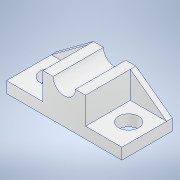
# Autodesk Inventor part: Part1
Saved by Autodesk Inventor 2022 (Build 260153000, 153)
## iProperties
Created: 2021-10-05
Part Number: Part1
Material: Aluminum 6061
Document SubType Name: Modeling
Designer: Lucas
Density: 2.7 g/cm^3
Appearance: Aluminum - Flat
Mass: 213.769 g
Surface Area: 180.738 cm^2
Volume: 79.1737 cm^3
Author: Lucas
Autodesk Inventor part; units mm, degrees
ref_plane "YZ Plane" through (0, 0, 0) normal (1, 0, 0) x (0, 1, 0)
ref_plane "XZ Plane" through (0, 0, 0) normal (0, 1, 0) x (-1, 0, 0)
ref_plane "XY Plane" through (0, 0, 0) normal (0, 0, 1) x (1, 0, 0)
sketch "Sketch1" plane through (0, 0, 0) normal (0, 0, 1) x (1, 0, 0)
  line L0 (-51.5, 0) -> (51.5, 0)
  line L1 (51.5, 0) -> (51.5, 10)
  line L2 (51.5, 10) -> (19, 10)
  line L3 (19, 10) -> (19, 34)
  line L4 (19, 34) -> (10, 34)
  arc A0 (-10, 34) -> (10, 34) centre (0, 34) ccw
  line L5 (-10, 34) -> (-19, 34)
  line L6 (-19, 34) -> (-19, 10)
  line L7 (-19, 10) -> (-51.5, 10)
  line L8 (-51.5, 10) -> (-51.5, 0)
  point P0 (0, 0)
  dimension "d0" = 103
  dimension "d4" = 38
  dimension "d6" = 34
  dimension "d7" = 10
  dimension "d8" = 51.5
  dimension "d9" = 0
  dimension "d10" = 10
  constraints: 18 end point, 4 perpendicular, 3 collinear, 3 point on line, 2 parallel, 2 point on circle, 2 vertical, 1 centre point
  measures "d0" distance of L0.start L0.end
  measures "d4" distance between parallel lines of L3 L6
  measures "d6" distance between parallel lines of L5 L0
  measures "d7" radius of A0
  measures "d8" distance from line of L8 point (0, 0)
  measures "d9" distance from line of L0 point (0, 0)
  measures "d10" distance of L7.end L0.start
extrude "Extrusion1" add sketch "Sketch1" along normal mid plane 45
sketch "Sketch2" plane through (0, 0, -22.5) normal (0, 0, -1) x (-1, 0, 0)
  line L0 (-19, 34) -> (-10, 34) projected
  line L1 (-19, 10) -> (-51.5, 10) projected
  line L2 (-19, 34) -> (-51.5, 10)
  line L3 (-19, 10) -> (-19, 34) projected
  line L4 (-51.5, 10) -> (-19, 10) projected
  line L5 (-19, 10) -> (-51.5, 10)
  point P0 (0, 0)
  constraints: 4 end point, 1 collinear
extrude "Extrusion2" add sketch "Sketch2" against normal blind 5
sketch "Sketch3" plane through (0, 0, -22.5) normal (0, 0, -1) x (-1, 0, 0)
  line L0 (19, 34) -> (19, 10) projected
  line L1 (19, 10) -> (51.5, 10) projected
  line L2 (19, 34) -> (51.5, 10)
  point P0 (0, 0)
  constraints: 2 end point
extrude "Extrusion3" add sketch "Sketch3" against normal blind 5
sketch "Sketch4" plane through (19, 10, 22.5) normal (0, 1, 0) x (1, 0, 0)
  line L0 (-38, 0) -> (-70.5, 0) projected
  line L1 (32.5, 0) -> (0, 0) projected
  line L2 (-70.5, 40) -> (-70.5, 0) projected
  point P0 (-19, 22.5)
  point P1 (16, 22.5)
  point P2 (-54, 22.5)
  dimension "d17" = 70
  dimension "d18" = 22.5
  dimension "d19" = 22.5
  dimension "d20" = 16.5
  measures "d17" distance of point (16, 22.5) point (-54, 22.5)
  measures "d18" distance from line of L0 point (-54, 22.5)
  measures "d19" distance from line of L1 point (16, 22.5)
  measures "d20" distance from line of L2 point (-54, 22.5)
hole "Hole1" at (35, 10, 0) at (-35, 10, 0) direction (0, -1, 0) diameter 18 end through all
ref_plane "Work Plane1" through (0, 0, -72.5) normal (0, 0, -1) x (-1, 0, 0)
sketch "Sketch5" plane through (0, 0, -72.5) normal (0, 0, -1) x (-1, 0, 0)
  line L0 (-10, 22) -> (10, 22) construction
  line L1 (10, 22) -> (10, 2) construction
  line L2 (10, 2) -> (-10, 2) construction
  line L3 (-10, 2) -> (-10, 22) construction
  line L4 (-51.5, 0) -> (51.5, 0) projected
  point P0 (0, 0)
  dimension "d34" = 20
  dimension "d40" = 2
  dimension "d44" = 10
  constraints: 2 other
  measures "d34" distance of L0.end L0.start
  measures "d40" distance between parallel lines of L4 L2
  measures "d44" horizontal distance of point (0, 0) L2.end
decal "Decal1"
sketch "Sketch6" plane through (0, 0, -72.5) normal (0, 0, -1) x (-1, 0, 0)
  line L0 (-46.7531, 9.3378) -> (-6.7156, 9.3378) construction
  line L1 (-6.7156, 9.3378) -> (-6.7156, 3.5407) construction
  line L2 (-6.7156, 3.5407) -> (-46.7531, 3.5407) construction
  line L3 (-46.7531, 3.5407) -> (-46.7531, 9.3378) construction
  line L4 (-46.2466, 4.115) -> (-46.2466, 9.115)
  line L5 (-46.2466, 9.115) -> (-43.1185, 9.115)
  line L6 (-43.1185, 9.115) -> (-43.1185, 8.5234)
  line L7 (-43.1185, 8.5234) -> (-45.5821, 8.5234)
  line L8 (-45.5821, 8.5234) -> (-45.5821, 7.1539)
  line L9 (-45.5821, 7.1539) -> (-43.2847, 7.1539)
  line L10 (-43.2847, 7.1539) -> (-43.2847, 6.5623)
  line L11 (-43.2847, 6.5623) -> (-45.5821, 6.5623)
  line L12 (-45.5821, 6.5623) -> (-45.5821, 4.7065)
  line L13 (-45.5821, 4.7065) -> (-43.1185, 4.7065)
  line L14 (-43.1185, 4.7065) -> (-43.1185, 4.115)
  line L15 (-43.1185, 4.115) -> (-46.2466, 4.115)
  spline S0 degree 2 poles (-40.4362, 4.0258) (-40.9224, 4.0258) (-41.7449, 4.354) (-42.0448, 4.6822) knots 0 0 0 1 2 2 2
  spline S1 degree 2 poles (-42.0448, 4.6822) (-42.3446, 5.0064) (-42.6728, 5.9788) (-42.6728, 6.6109) knots 0 0 0 1 2 2 2
  spline S2 degree 2 poles (-42.6728, 6.6109) (-42.6728, 7.239) (-42.3527, 8.1709) (-42.0488, 8.5153) knots 0 0 0 1 2 2 2
  spline S3 degree 2 poles (-42.0488, 8.5153) (-41.749, 8.8516) (-40.9305, 9.2041) (-40.424, 9.2041) knots 0 0 0 1 2 2 2
  spline S4 degree 2 poles (-40.424, 9.2041) (-40.1728, 9.2041) (-39.7312, 9.1312) (-39.5448, 9.0744) knots 0 0 0 1 2 2 2
  spline S5 degree 2 poles (-39.5448, 9.0744) (-39.3827, 9.0218) (-39.0464, 8.8719) (-38.8803, 8.7827) knots 0 0 0 1 2 2 2
  line L16 (-38.8803, 8.7827) -> (-38.8803, 7.9804)
  line L17 (-38.8803, 7.9804) -> (-38.933, 7.9804)
  spline S6 degree 2 poles (-38.933, 7.9804) (-39.0221, 8.0615) (-39.2976, 8.2884) (-39.4962, 8.3978) knots 0 0 0 1 2 2 2
  spline S7 degree 2 poles (-39.4962, 8.3978) (-39.6866, 8.5031) (-40.1364, 8.6368) (-40.4281, 8.6368) knots 0 0 0 1 2 2 2
  spline S8 degree 2 poles (-40.4281, 8.6368) (-40.7482, 8.6368) (-41.3195, 8.3735) (-41.5343, 8.1223) knots 0 0 0 1 2 2 2
  spline S9 degree 2 poles (-41.5343, 8.1223) (-41.7449, 7.867) (-41.98, 7.0931) (-41.98, 6.6109) knots 0 0 0 1 2 2 2
  spline S10 degree 2 poles (-41.98, 6.6109) (-41.98, 6.0963) (-41.7328, 5.3548) (-41.518, 5.0996) knots 0 0 0 1 2 2 2
  spline S11 degree 2 poles (-41.518, 5.0996) (-41.3073, 4.8524) (-40.7441, 4.6012) (-40.4281, 4.6012) knots 0 0 0 1 2 2 2
  spline S12 degree 2 poles (-40.4281, 4.6012) (-40.1404, 4.6012) (-39.6501, 4.743) (-39.4597, 4.8484) knots 0 0 0 1 2 2 2
  spline S13 degree 2 poles (-39.4597, 4.8484) (-39.2774, 4.9537) (-39.0059, 5.1725) (-38.9289, 5.2495) knots 0 0 0 1 2 2 2
  line L18 (-38.9289, 5.2495) -> (-38.8803, 5.2495)
  line L19 (-38.8803, 5.2495) -> (-38.8803, 4.4553)
  spline S14 degree 2 poles (-38.8803, 4.4553) (-39.0464, 4.3783) (-39.3381, 4.2365) (-39.5448, 4.1717) knots 0 0 0 1 2 2 2
  spline S15 degree 2 poles (-39.5448, 4.1717) (-39.7636, 4.0988) (-40.1364, 4.0258) (-40.4362, 4.0258) knots 0 0 0 1 2 2 2
  line L20 (-35.3187, 4.115) -> (-38.4022, 4.115)
  line L21 (-38.4022, 4.115) -> (-38.4022, 4.824)
  spline S16 degree 2 poles (-38.4022, 4.824) (-38.0699, 5.136) (-37.4783, 5.7155) (-37.1947, 6.0274) knots 0 0 0 1 2 2 2
  spline S17 degree 2 poles (-37.1947, 6.0274) (-36.6234, 6.6555) (-36.2061, 7.4091) (-36.2061, 7.8103) knots 0 0 0 1 2 2 2
  spline S18 degree 2 poles (-36.2061, 7.8103) (-36.2061, 8.021) (-36.3357, 8.337) (-36.4532, 8.4383) knots 0 0 0 1 2 2 2
  spline S19 degree 2 poles (-36.4532, 8.4383) (-36.5707, 8.5396) (-36.8787, 8.6409) (-37.065, 8.6409) knots 0 0 0 1 2 2 2
  spline S20 degree 2 poles (-37.065, 8.6409) (-37.2433, 8.6409) (-37.608, 8.5518) (-37.7741, 8.4829) knots 0 0 0 1 2 2 2
  spline S21 degree 2 poles (-37.7741, 8.4829) (-37.9159, 8.4261) (-38.1793, 8.2641) (-38.2603, 8.2073) knots 0 0 0 1 2 2 2
  line L22 (-38.2603, 8.2073) -> (-38.2968, 8.2073)
  line L23 (-38.2968, 8.2073) -> (-38.2968, 8.9205)
  spline S22 degree 2 poles (-38.2968, 8.9205) (-38.0902, 9.0218) (-37.3487, 9.2203) (-37.0164, 9.2203) knots 0 0 0 1 2 2 2
  spline S23 degree 2 poles (-37.0164, 9.2203) (-36.3155, 9.2203) (-35.5253, 8.4788) (-35.5253, 7.8467) knots 0 0 0 1 2 2 2
  spline S24 degree 2 poles (-35.5253, 7.8467) (-35.5253, 7.5509) (-35.6631, 7.0566) (-35.7847, 6.8459) knots 0 0 0 1 2 2 2
  spline S25 degree 2 poles (-35.7847, 6.8459) (-35.9062, 6.6271) (-36.2587, 6.1976) (-36.4532, 5.991) knots 0 0 0 1 2 2 2
  spline S26 degree 2 poles (-36.4532, 5.991) (-36.7693, 5.6466) (-37.5432, 4.9091) (-37.7741, 4.6944) knots 0 0 0 1 2 2 2
  line L24 (-37.7741, 4.6944) -> (-35.3187, 4.6944)
  line L25 (-35.3187, 4.6944) -> (-35.3187, 4.115)
  line L26 (-30.6712, 5.9991) -> (-32.5634, 5.9991)
  line L27 (-32.5634, 5.9991) -> (-32.5634, 6.6069)
  line L28 (-32.5634, 6.6069) -> (-30.6712, 6.6069)
  line L29 (-30.6712, 6.6069) -> (-30.6712, 5.9991)
  line L30 (-24.7757, 4.115) -> (-27.8592, 4.115)
  line L31 (-27.8592, 4.115) -> (-27.8592, 4.824)
  spline S27 degree 2 poles (-27.8592, 4.824) (-27.527, 5.136) (-26.9354, 5.7155) (-26.6518, 6.0274) knots 0 0 0 1 2 2 2
  spline S28 degree 2 poles (-26.6518, 6.0274) (-26.0804, 6.6555) (-25.6631, 7.4091) (-25.6631, 7.8103) knots 0 0 0 1 2 2 2
  spline S29 degree 2 poles (-25.6631, 7.8103) (-25.6631, 8.021) (-25.7928, 8.337) (-25.9103, 8.4383) knots 0 0 0 1 2 2 2
  spline S30 degree 2 poles (-25.9103, 8.4383) (-26.0278, 8.5396) (-26.3357, 8.6409) (-26.5221, 8.6409) knots 0 0 0 1 2 2 2
  spline S31 degree 2 poles (-26.5221, 8.6409) (-26.7004, 8.6409) (-27.065, 8.5518) (-27.2312, 8.4829) knots 0 0 0 1 2 2 2
  spline S32 degree 2 poles (-27.2312, 8.4829) (-27.373, 8.4261) (-27.6364, 8.2641) (-27.7174, 8.2073) knots 0 0 0 1 2 2 2
  line L32 (-27.7174, 8.2073) -> (-27.7539, 8.2073)
  line L33 (-27.7539, 8.2073) -> (-27.7539, 8.9205)
  spline S33 degree 2 poles (-27.7539, 8.9205) (-27.5472, 9.0218) (-26.8057, 9.2203) (-26.4735, 9.2203) knots 0 0 0 1 2 2 2
  spline S34 degree 2 poles (-26.4735, 9.2203) (-25.7725, 9.2203) (-24.9824, 8.4788) (-24.9824, 7.8467) knots 0 0 0 1 2 2 2
  spline S35 degree 2 poles (-24.9824, 7.8467) (-24.9824, 7.5509) (-25.1202, 7.0566) (-25.2417, 6.8459) knots 0 0 0 1 2 2 2
  spline S36 degree 2 poles (-25.2417, 6.8459) (-25.3633, 6.6271) (-25.7158, 6.1976) (-25.9103, 5.991) knots 0 0 0 1 2 2 2
  spline S37 degree 2 poles (-25.9103, 5.991) (-26.2263, 5.6466) (-27.0002, 4.9091) (-27.2312, 4.6944) knots 0 0 0 1 2 2 2
  line L34 (-27.2312, 4.6944) -> (-24.7757, 4.6944)
  line L35 (-24.7757, 4.6944) -> (-24.7757, 4.115)
  line L36 (-21.2749, 4.115) -> (-23.7142, 4.115)
  line L37 (-23.7142, 4.115) -> (-23.7142, 4.6255)
  line L38 (-23.7142, 4.6255) -> (-22.8065, 4.6255)
  line L39 (-22.8065, 4.6255) -> (-22.8065, 7.9764)
  line L40 (-22.8065, 7.9764) -> (-23.7142, 7.9764)
  line L41 (-23.7142, 7.9764) -> (-23.7142, 8.4343)
  spline S38 degree 2 poles (-23.7142, 8.4343) (-23.1996, 8.4343) (-22.7133, 8.726) (-22.6809, 9.1312) knots 0 0 0 1 2 2 2
  line L42 (-22.6809, 9.1312) -> (-22.1623, 9.1312)
  line L43 (-22.1623, 9.1312) -> (-22.1623, 4.6255)
  line L44 (-22.1623, 4.6255) -> (-21.2749, 4.6255)
  line L45 (-21.2749, 4.6255) -> (-21.2749, 4.115)
  line L46 (-18.2766, 9.3378) -> (-20.2336, 3.0291)
  line L47 (-20.2336, 3.0291) -> (-20.8009, 3.0291)
  line L48 (-20.8009, 3.0291) -> (-18.8519, 9.3378)
  line L49 (-18.8519, 9.3378) -> (-18.2766, 9.3378)
  line L50 (-14.642, 4.115) -> (-17.7255, 4.115)
  line L51 (-17.7255, 4.115) -> (-17.7255, 4.824)
  spline S39 degree 2 poles (-17.7255, 4.824) (-17.3932, 5.136) (-16.8017, 5.7155) (-16.518, 6.0274) knots 0 0 0 1 2 2 2
  spline S40 degree 2 poles (-16.518, 6.0274) (-15.9467, 6.6555) (-15.5294, 7.4091) (-15.5294, 7.8103) knots 0 0 0 1 2 2 2
  spline S41 degree 2 poles (-15.5294, 7.8103) (-15.5294, 8.021) (-15.6591, 8.337) (-15.7766, 8.4383) knots 0 0 0 1 2 2 2
  spline S42 degree 2 poles (-15.7766, 8.4383) (-15.8941, 8.5396) (-16.202, 8.6409) (-16.3884, 8.6409) knots 0 0 0 1 2 2 2
  spline S43 degree 2 poles (-16.3884, 8.6409) (-16.5667, 8.6409) (-16.9313, 8.5518) (-17.0975, 8.4829) knots 0 0 0 1 2 2 2
  spline S44 degree 2 poles (-17.0975, 8.4829) (-17.2393, 8.4261) (-17.5026, 8.2641) (-17.5837, 8.2073) knots 0 0 0 1 2 2 2
  line L52 (-17.5837, 8.2073) -> (-17.6202, 8.2073)
  line L53 (-17.6202, 8.2073) -> (-17.6202, 8.9205)
  spline S45 degree 2 poles (-17.6202, 8.9205) (-17.4135, 9.0218) (-16.672, 9.2203) (-16.3398, 9.2203) knots 0 0 0 1 2 2 2
  spline S46 degree 2 poles (-16.3398, 9.2203) (-15.6388, 9.2203) (-14.8487, 8.4788) (-14.8487, 7.8467) knots 0 0 0 1 2 2 2
  spline S47 degree 2 poles (-14.8487, 7.8467) (-14.8487, 7.5509) (-14.9864, 7.0566) (-15.108, 6.8459) knots 0 0 0 1 2 2 2
  spline S48 degree 2 poles (-15.108, 6.8459) (-15.2296, 6.6271) (-15.5821, 6.1976) (-15.7766, 5.991) knots 0 0 0 1 2 2 2
  spline S49 degree 2 poles (-15.7766, 5.991) (-16.0926, 5.6466) (-16.8665, 4.9091) (-17.0975, 4.6944) knots 0 0 0 1 2 2 2
  line L54 (-17.0975, 4.6944) -> (-14.642, 4.6944)
  line L55 (-14.642, 4.6944) -> (-14.642, 4.115)
  point P0 (0, 0)
  constraints: 2 other
emboss "Emboss1" sketch "Sketch6" operation add depth 1 direction (0, 0, 1)
equation "\"d8\" = 0.5 * d0"
equation "\"d44\" = 0.5 * d34"
body "Solid1"
